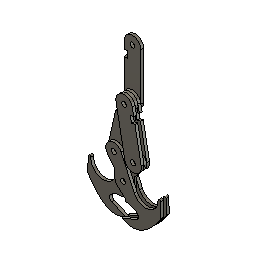
Gravitational Hook (Autodesk Fusion 360 design; units mm, degrees)
part number: 2026-08-22-10-27-55-705
part number: 2026-08-22-15-39-22-120
part number: 2026-08-22-15-42-42-149
part number: 2026-08-22-15-56-56-558
part number: 2026-08-22-15-58-14-669
Autodesk Fusion 360 part; units mm, degrees
sketch "Sketch2" plane through (0, 0, 0) normal (0, 0, 1) x (1, 0, 0)
  circle A0 centre (0.875, 0) radius 0.875
  circle A1 centre (10.75, -0.0061) radius 9
  line L0 (0, 0) -> (0, 10.5)
  spline S0 degree 5 poles (0, 10.5) (0.3351, 10.9779) (1.0082, 11.9189) (2.0267, 13.2858) (3.4027, 15.0183) (5.1533, 17.0285) (6.9356, 18.8737) (8.7506, 20.5401) (10.599, 22.0098) (12.4805, 23.2619) (14.3936, 24.2733) (16.3362, 25.021) (18.306, 25.4844) (20.3008, 25.6483) (22.3185, 25.5085) (24.3575, 25.0691) (26.0048, 24.4839) (27.249, 23.9165) (28.0824, 23.4816) (28.5, 23.25) knots 0 0 0 0 0 0 0.066667 0.133333 0.2 0.266667 0.333333 0.4 0.466667 0.533333 0.6 0.666667 0.733333 0.8 0.866667 0.933333 1 1 1 1 1 1
  circle A2 centre (18.75, 16.9939) radius 2.5
  line L1 (28.5, 23.25) -> (17.8858, 19.3398)
  arc A3 (16.9675, 15.241) -> (25.75, 11.9939) centre (24.8106, 22.9537) ccw
  line L2 (25.75, 11.9939) -> (25.75, 9.9939)
  line L3 (25.75, 9.9939) -> (32.821, 2.9228)
  line L4 (25.75, 9.9939) -> (15.75, 9.9939) construction
  line L5 (32.821, 2.9228) -> (32.821, -5.0772)
  circle A4 centre (33.25, -15.5061) radius 1.75
  circle A5 centre (33.25, -15.5061) radius 5.75
  line L6 (32.821, -5.0772) -> (37.9146, -12.144)
  line L7 (19.049, 3.4763) -> (27.9479, -17.731)
  line L8 (81.3303, -10.3713) -> (81.3303, 23.6287)
  arc A6 (81.3303, 23.6287) -> (69.3303, 23.6287) centre (75.3303, 23.6287) ccw
  line L9 (69.3303, 23.6287) -> (69.3303, -10.3713)
  arc A7 (69.3303, -10.3713) -> (81.3303, -10.3713) centre (75.3303, -10.3713) ccw
  line L10 (75.3303, -10.3713) -> (75.3303, 23.6287) construction
  circle A8 centre (75.3303, 23.6287) radius 1.75
  circle A9 centre (75.3303, -10.3713) radius 1.75
  line L11 (69.3303, 18.1287) -> (71.8303, 18.1287)
  line L12 (71.8303, 18.1287) -> (71.8303, 13.6287)
  line L13 (71.8303, 13.6287) -> (69.3303, 13.6287)
  line L14 (69.3303, 13.6287) -> (69.3303, 18.1287)
  circle A10 centre (27, 0) radius 1.75
  point P0 (10, 21.5)
  point P1 (19, 25.5)
  dimension "d1" = 1.75
  dimension "d2" = 18
  dimension "d3" = 10.5
  dimension "d4" = 11
  dimension "d5" = 10
  dimension "d6" = 9
  dimension "d7" = 4
  dimension "d8" = 2.25
  dimension "d9" = 9.5
  dimension "d10" = 5
  dimension "d11" = 17
  dimension "d12" = 8
  dimension "d13" = 5
  dimension "d14" = 7
  dimension "d15" = 11
  dimension "d16" = 2
  dimension "d17" = 10
  dimension "d18" = 135
  dimension "d19" = 8
  dimension "d20" = 3.5
  dimension "d21" = 11.5
  dimension "d22" = 22.5
  dimension "d23" = 15.5
  dimension "d24" = 34
  dimension "d25" = 12
  dimension "d26" = 3.5
  dimension "d27" = 3.5
  dimension "d28" = 2.5
  dimension "d29" = 4.5
  dimension "d30" = 5.5
  dimension "d31" = 3.5
  dimension "d32" = 27
  constraint coincident L0.start A0
  constraint coincident L0.start origin
  constraint vertical L0
  constraint coincident A2 L1.end
  constraint tangent A2 L1
  constraint coincident A2 A3.start
  constraint tangent A2 A3
  constraint vertical L2
  constraint horizontal L4
  constraint parallel L2 L5
  constraint concentric A4 A5
  constraint coincident A5 L6.end
  constraint tangent A5 L6
  constraint coincident A1 L7.start
  constraint coincident A5 L7.end
  constraint tangent A5 L7
  constraint tangent A1 L7
  constraint tangent L8 A6
  constraint tangent A6 L9
  constraint parallel L8 L9
  constraint tangent L9 A7
  constraint tangent L8 A7
  constraint vertical L10
  constraint concentric A6 A8
  constraint concentric A7 A9
  constraint horizontal L11
  constraint vertical L12
  constraint horizontal L13
  constraint vertical L14
  constraint coincident L9 L11.start
  measures "d1" diameter of A0
  measures "d2" diameter of A1
  measures "d3" distance of L0.start L0.end
  measures "d4" vertical distance of L0.end P0
  measures "d5" horizontal distance of L0.end P0
  measures "d6" horizontal distance of P0 P1
  measures "d7" vertical distance of P0 P1
  measures "d8" distance of P1 S0.end
  measures "d9" distance of P1 S0.end
  measures "d10" diameter of A2
  measures "d11" vertical distance of A1.centre A2.centre
  measures "d12" horizontal distance of A1.centre A2.centre
  measures "d13" vertical distance of A2.centre A3.end
  measures "d14" horizontal distance of A2.centre A3.end
  measures "d15" radius of A3
  measures "d16" distance of A3.end L2.end
  measures "d17" distance of L2.end L3.end
  measures "d18" angle of L3 L4
  measures "d19" distance of L3.end L5.end
  measures "d20" diameter of A4
  measures "d21" diameter of A5
  measures "d22" horizontal distance of A1.centre A4.centre
  measures "d23" vertical distance of A1.centre A4.centre
  measures "d24" distance of A7.centre A6.centre
  measures "d25" diameter of A6
  measures "d26" diameter of A8
  measures "d27" diameter of A9
  measures "d28" distance of L11.start L11.end
  measures "d29" distance of L11.start L13.end
  measures "d30" distance of A6.centre L11
  measures "d31" diameter of A10
  measures "d32" distance of L0.start A10.centre
extrude "Extrude1" add sketch "Sketch2" along normal mid plane 2 contours A0 | A0 A1 L0 S0 A2 L1 A3 L2 L3 L5 A5 L6 L7 | A5 makes body 1 in component "Hook"
extrude "Extrude1'" add sketch "Sketch2" along normal mid plane 2 separate body contours L8 A6 L9 A7 L11 L12 L13 makes body 2 in component "Link"
extrude "Extrude1''" add sketch "Sketch2" along normal mid plane 2 separate body contours A0 | A0 A1 L0 S0 A2 L1 A3 L2 L3 L5 A5 L6 L7 | A5 makes body 3 in component "Hook 2"
extrude "Extrude1'''" add sketch "Sketch2" along normal mid plane 2 separate body contours A0 | A0 A1 L0 S0 A2 L1 A3 L2 L3 L5 A5 L6 L7 | A5 makes body 4 in component "Hook 3"
pattern_linear "00000000-0000-0000-0000-000000000000" [suppressed]
component "Link" placed x (0.960202, -0.279307, 0) y (0.279307, 0.960202, 0) z (0, 0, 1) at (-48.6855, 46.5049, 2)
component "Hook" placed x (-1, 0, 0) y (0, -1, 0) z (0, 0, 1) at (54, 0, 0)
component "Hook 2" placed x (-1, 0, 0) y (0, -1, 0) z (0, 0, 1) at (54, 0, 4)
component "Hook 3" placed x (0.99095, -0.13423, 0) y (-0.13423, -0.99095, 0) z (0, 0, -1) at (0.2443, 3.6242, 2)
component "Link" placed x (-0.989004, -0.147892, 0) y (-0.147892, 0.989004, 0) z (0, 0, -1) at (108.2429, 35.9248, 4)
component "Link" placed x (-0.989004, -0.147892, 0) y (-0.147892, 0.989004, 0) z (0, 0, -1) at (108.2429, 35.9248, 0)
component "Link" placed x (1, 0, 0) y (0, 1, 0) z (0, 0, 1) at (-45.0839, 58.5243, -2)
